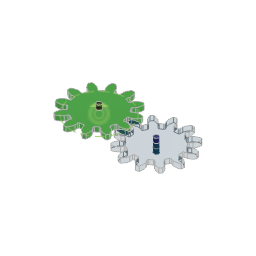
simple_gear_power (Autodesk Fusion 360 design; units mm, degrees)
description: Spur Gear; Module: 10.0; Num Teeth: 12; Pressure Angle: 20.0; Backlash: 0.00 mm
part number: 2026-04-30-14-06-16-626
part number: 2026-04-30-14-27-06-127
part number: 2026-04-30-14-27-10-473
part number: 2026-04-30-14-27-12-573
part number: 2026-04-30-14-27-14-794
Autodesk Fusion 360 part; units mm, degrees
(part 1 of 2)
sketch "Base Circle" plane through (0, 0, 0) normal (0, 0, 1) x (1, 0, 0)
  circle A0 centre (0, 0) radius 48.43
  circle A1 centre (0, 0) radius 5
extrude "Extrude5" add sketch "Base Circle" along normal blind 10 makes body 1
sketch "Gear Tooth" plane through (0, 0, 0) normal (0, 0, 1) x (1, 0, 0)
  spline S0 degree 5 poles (55.7833, -8.1916) (55.824, -8.1975) (55.9054, -8.2082) (56.0278, -8.2201) (56.1916, -8.2285) (56.3971, -8.2288) (56.6031, -8.2218) (56.8094, -8.2105) (57.0158, -8.1967) (57.2224, -8.1814) (57.429, -8.1642) (57.6357, -8.1445) (57.8425, -8.1217) (58.0493, -8.0952) (58.2562, -8.0651) (58.4632, -8.0317) (58.6701, -7.9955) (58.877, -7.957) (59.0839, -7.9164) (59.2907, -7.8739) (59.4973, -7.8293) (59.7039, -7.7827) (59.9104, -7.7337) (60.1168, -7.6825) (60.3231, -7.6291) (60.5293, -7.5736) (60.7353, -7.516) (60.9412, -7.4565) (61.1469, -7.3952) (61.3524, -7.332) (61.5578, -7.267) (61.7629, -7.2001) (61.9679, -7.1315) (62.1727, -7.061) (62.3773, -6.9888) (62.5816, -6.9148) (62.7857, -6.839) (62.9896, -6.7616) (63.1933, -6.6825) (63.3967, -6.6018) (63.5998, -6.5195) (63.8027, -6.4355) (64.0053, -6.3499) (64.2077, -6.2628) (64.4097, -6.174) (64.6115, -6.0837) (64.813, -5.9919) (65.0142, -5.8985) (65.2151, -5.8037) (65.4157, -5.7073) (65.616, -5.6095) (65.8159, -5.5101) (66.0155, -5.4094) (66.2148, -5.3071) (66.4138, -5.2035) (66.6124, -5.0984) (66.8106, -4.9919) (67.0085, -4.884) (67.2061, -4.7747) (67.4033, -4.664) (67.6001, -4.552) (67.7965, -4.4385) (67.9926, -4.3238) (68.1883, -4.2077) (68.3835, -4.0902) (68.5784, -3.9715) (68.7729, -3.8514) (68.967, -3.73) (69.1607, -3.6073) (69.354, -3.4834) (69.5468, -3.3581) (69.7008, -3.2569) (69.816, -3.1804) (69.8928, -3.1292) (69.9312, -3.1035) knots 0 0 0 0 0 0 0.01428571 0.02857143 0.04285714 0.05714286 0.07142857 0.08571429 0.1 0.11428571 0.12857143 0.14285714 0.15714286 0.17142857 0.18571429 0.2 0.21428571 0.22857143 0.24285714 0.25714286 0.27142857 0.28571429 0.3 0.31428571 0.32857143 0.34285714 0.35714286 0.37142857 0.38571429 0.4 0.41428571 0.42857143 0.44285714 0.45714286 0.47142857 0.48571429 0.5 0.51428571 0.52857143 0.54285714 0.55714286 0.57142857 0.58571429 0.6 0.61428571 0.62857143 0.64285714 0.65714286 0.67142857 0.68571429 0.7 0.71428571 0.72857143 0.74285714 0.75714286 0.77142857 0.78571429 0.8 0.81428571 0.82857143 0.84285714 0.85714286 0.87142857 0.88571429 0.9 0.91428571 0.92857143 0.94285714 0.95714286 0.97142857 0.98571429 1 1 1 1 1 1
  spline S1 degree 5 poles (55.7833, 8.1916) (55.824, 8.1975) (55.9054, 8.2082) (56.0278, 8.2201) (56.1916, 8.2285) (56.3971, 8.2288) (56.6031, 8.2218) (56.8094, 8.2105) (57.0158, 8.1967) (57.2224, 8.1814) (57.429, 8.1642) (57.6357, 8.1445) (57.8425, 8.1217) (58.0493, 8.0952) (58.2562, 8.0651) (58.4632, 8.0317) (58.6701, 7.9955) (58.877, 7.957) (59.0839, 7.9164) (59.2907, 7.8739) (59.4973, 7.8293) (59.7039, 7.7827) (59.9104, 7.7337) (60.1168, 7.6825) (60.3231, 7.6291) (60.5293, 7.5736) (60.7353, 7.516) (60.9412, 7.4565) (61.1469, 7.3952) (61.3524, 7.332) (61.5578, 7.267) (61.7629, 7.2001) (61.9679, 7.1315) (62.1727, 7.061) (62.3773, 6.9888) (62.5816, 6.9148) (62.7857, 6.839) (62.9896, 6.7616) (63.1933, 6.6825) (63.3967, 6.6018) (63.5998, 6.5195) (63.8027, 6.4355) (64.0053, 6.3499) (64.2077, 6.2628) (64.4097, 6.174) (64.6115, 6.0837) (64.813, 5.9919) (65.0142, 5.8985) (65.2151, 5.8037) (65.4157, 5.7073) (65.616, 5.6095) (65.8159, 5.5101) (66.0155, 5.4094) (66.2148, 5.3071) (66.4138, 5.2035) (66.6124, 5.0984) (66.8106, 4.9919) (67.0085, 4.884) (67.2061, 4.7747) (67.4033, 4.664) (67.6001, 4.552) (67.7965, 4.4385) (67.9926, 4.3238) (68.1883, 4.2077) (68.3835, 4.0902) (68.5784, 3.9715) (68.7729, 3.8514) (68.967, 3.73) (69.1607, 3.6073) (69.354, 3.4834) (69.5468, 3.3581) (69.7008, 3.2569) (69.816, 3.1804) (69.8928, 3.1292) (69.9312, 3.1035) knots 0 0 0 0 0 0 0.01428571 0.02857143 0.04285714 0.05714286 0.07142857 0.08571429 0.1 0.11428571 0.12857143 0.14285714 0.15714286 0.17142857 0.18571429 0.2 0.21428571 0.22857143 0.24285714 0.25714286 0.27142857 0.28571429 0.3 0.31428571 0.32857143 0.34285714 0.35714286 0.37142857 0.38571429 0.4 0.41428571 0.42857143 0.44285714 0.45714286 0.47142857 0.48571429 0.5 0.51428571 0.52857143 0.54285714 0.55714286 0.57142857 0.58571429 0.6 0.61428571 0.62857143 0.64285714 0.65714286 0.67142857 0.68571429 0.7 0.71428571 0.72857143 0.74285714 0.75714286 0.77142857 0.78571429 0.8 0.81428571 0.82857143 0.84285714 0.85714286 0.87142857 0.88571429 0.9 0.91428571 0.92857143 0.94285714 0.95714286 0.97142857 0.98571429 1 1 1 1 1 1
  arc A0 (69.9312, -3.1035) -> (69.9312, 3.1035) centre (0, 0) ccw
  line L0 (47.9062, -7.0348) -> (55.7833, -8.1916)
  line L1 (47.9062, 7.0348) -> (55.7833, 8.1916)
  line L2 (47.9062, -7.0348) -> (47.9062, 7.0348)
  point P0 (56.7633, -8.2126)
  point P1 (57.7576, -8.1306)
  point P2 (58.7606, -7.9784)
  point P3 (59.77, -7.7667)
  point P4 (60.7841, -7.5016)
  point P5 (61.8016, -7.1869)
  point P6 (62.8211, -6.8253)
  point P7 (63.8417, -6.4188)
  point P8 (64.8622, -5.9688)
  point P9 (65.8818, -5.4767)
  point P10 (66.8994, -4.9433)
  point P11 (67.9141, -4.3695)
  point P12 (68.925, -3.756)
  point P13 (56.7633, 8.2126)
  point P14 (57.7576, 8.1306)
  point P15 (58.7606, 7.9784)
  point P16 (59.77, 7.7667)
  point P17 (60.7841, 7.5016)
  point P18 (61.8016, 7.1869)
  point P19 (62.8211, 6.8253)
  point P20 (63.8417, 6.4188)
  point P21 (64.8622, 5.9688)
  point P22 (65.8818, 5.4767)
  point P23 (66.8994, 4.9433)
  point P24 (67.9141, 4.3695)
  point P25 (68.925, 3.756)
extrude "Extrude6" add sketch "Gear Tooth" along normal blind 10 bodies 1
fillet "Fillet3" radius 2 2 edges at (47.9161, -7.0363, 5) (47.9161, 7.0363, 5) on bodies 1
pattern_circular "C-Pattern3" count 12 over 360 about axis through (0, 0, 0) along (0, 0, 1) of "Extrude6", "Fillet3"
sketch "Diametrial Pitch Circle" plane through (0, 0, 0) normal (0, 0, 1) x (1, 0, 0)
  circle A0 centre (0, 0) radius 60 construction
sketch "Base Circle (1)" plane through (0, 0, 0) normal (0, 0, 1) x (1, 0, 0)
  circle A0 centre (0, 0) radius 48.43
  circle A1 centre (0, 0) radius 5
extrude "Extrude7" add sketch "Base Circle (1)" along normal blind 10 separate body makes body 2
sketch "Gear Tooth (1)" plane through (0, 0, 0) normal (0, 0, 1) x (1, 0, 0)
  spline S0 degree 5 poles (55.7833, -8.1916) (55.824, -8.1975) (55.9054, -8.2082) (56.0278, -8.2201) (56.1916, -8.2285) (56.3971, -8.2288) (56.6031, -8.2218) (56.8094, -8.2105) (57.0158, -8.1967) (57.2224, -8.1814) (57.429, -8.1642) (57.6357, -8.1445) (57.8425, -8.1217) (58.0493, -8.0952) (58.2562, -8.0651) (58.4632, -8.0317) (58.6701, -7.9955) (58.877, -7.957) (59.0839, -7.9164) (59.2907, -7.8739) (59.4973, -7.8293) (59.7039, -7.7827) (59.9104, -7.7337) (60.1168, -7.6825) (60.3231, -7.6291) (60.5293, -7.5736) (60.7353, -7.516) (60.9412, -7.4565) (61.1469, -7.3952) (61.3524, -7.332) (61.5578, -7.267) (61.7629, -7.2001) (61.9679, -7.1315) (62.1727, -7.061) (62.3773, -6.9888) (62.5816, -6.9148) (62.7857, -6.839) (62.9896, -6.7616) (63.1933, -6.6825) (63.3967, -6.6018) (63.5998, -6.5195) (63.8027, -6.4355) (64.0053, -6.3499) (64.2077, -6.2628) (64.4097, -6.174) (64.6115, -6.0837) (64.813, -5.9919) (65.0142, -5.8985) (65.2151, -5.8037) (65.4157, -5.7073) (65.616, -5.6095) (65.8159, -5.5101) (66.0155, -5.4094) (66.2148, -5.3071) (66.4138, -5.2035) (66.6124, -5.0984) (66.8106, -4.9919) (67.0085, -4.884) (67.2061, -4.7747) (67.4033, -4.664) (67.6001, -4.552) (67.7965, -4.4385) (67.9926, -4.3238) (68.1883, -4.2077) (68.3835, -4.0902) (68.5784, -3.9715) (68.7729, -3.8514) (68.967, -3.73) (69.1607, -3.6073) (69.354, -3.4834) (69.5468, -3.3581) (69.7008, -3.2569) (69.816, -3.1804) (69.8928, -3.1292) (69.9312, -3.1035) knots 0 0 0 0 0 0 0.01428571 0.02857143 0.04285714 0.05714286 0.07142857 0.08571429 0.1 0.11428571 0.12857143 0.14285714 0.15714286 0.17142857 0.18571429 0.2 0.21428571 0.22857143 0.24285714 0.25714286 0.27142857 0.28571429 0.3 0.31428571 0.32857143 0.34285714 0.35714286 0.37142857 0.38571429 0.4 0.41428571 0.42857143 0.44285714 0.45714286 0.47142857 0.48571429 0.5 0.51428571 0.52857143 0.54285714 0.55714286 0.57142857 0.58571429 0.6 0.61428571 0.62857143 0.64285714 0.65714286 0.67142857 0.68571429 0.7 0.71428571 0.72857143 0.74285714 0.75714286 0.77142857 0.78571429 0.8 0.81428571 0.82857143 0.84285714 0.85714286 0.87142857 0.88571429 0.9 0.91428571 0.92857143 0.94285714 0.95714286 0.97142857 0.98571429 1 1 1 1 1 1
  spline S1 degree 5 poles (55.7833, 8.1916) (55.824, 8.1975) (55.9054, 8.2082) (56.0278, 8.2201) (56.1916, 8.2285) (56.3971, 8.2288) (56.6031, 8.2218) (56.8094, 8.2105) (57.0158, 8.1967) (57.2224, 8.1814) (57.429, 8.1642) (57.6357, 8.1445) (57.8425, 8.1217) (58.0493, 8.0952) (58.2562, 8.0651) (58.4632, 8.0317) (58.6701, 7.9955) (58.877, 7.957) (59.0839, 7.9164) (59.2907, 7.8739) (59.4973, 7.8293) (59.7039, 7.7827) (59.9104, 7.7337) (60.1168, 7.6825) (60.3231, 7.6291) (60.5293, 7.5736) (60.7353, 7.516) (60.9412, 7.4565) (61.1469, 7.3952) (61.3524, 7.332) (61.5578, 7.267) (61.7629, 7.2001) (61.9679, 7.1315) (62.1727, 7.061) (62.3773, 6.9888) (62.5816, 6.9148) (62.7857, 6.839) (62.9896, 6.7616) (63.1933, 6.6825) (63.3967, 6.6018) (63.5998, 6.5195) (63.8027, 6.4355) (64.0053, 6.3499) (64.2077, 6.2628) (64.4097, 6.174) (64.6115, 6.0837) (64.813, 5.9919) (65.0142, 5.8985) (65.2151, 5.8037) (65.4157, 5.7073) (65.616, 5.6095) (65.8159, 5.5101) (66.0155, 5.4094) (66.2148, 5.3071) (66.4138, 5.2035) (66.6124, 5.0984) (66.8106, 4.9919) (67.0085, 4.884) (67.2061, 4.7747) (67.4033, 4.664) (67.6001, 4.552) (67.7965, 4.4385) (67.9926, 4.3238) (68.1883, 4.2077) (68.3835, 4.0902) (68.5784, 3.9715) (68.7729, 3.8514) (68.967, 3.73) (69.1607, 3.6073) (69.354, 3.4834) (69.5468, 3.3581) (69.7008, 3.2569) (69.816, 3.1804) (69.8928, 3.1292) (69.9312, 3.1035) knots 0 0 0 0 0 0 0.01428571 0.02857143 0.04285714 0.05714286 0.07142857 0.08571429 0.1 0.11428571 0.12857143 0.14285714 0.15714286 0.17142857 0.18571429 0.2 0.21428571 0.22857143 0.24285714 0.25714286 0.27142857 0.28571429 0.3 0.31428571 0.32857143 0.34285714 0.35714286 0.37142857 0.38571429 0.4 0.41428571 0.42857143 0.44285714 0.45714286 0.47142857 0.48571429 0.5 0.51428571 0.52857143 0.54285714 0.55714286 0.57142857 0.58571429 0.6 0.61428571 0.62857143 0.64285714 0.65714286 0.67142857 0.68571429 0.7 0.71428571 0.72857143 0.74285714 0.75714286 0.77142857 0.78571429 0.8 0.81428571 0.82857143 0.84285714 0.85714286 0.87142857 0.88571429 0.9 0.91428571 0.92857143 0.94285714 0.95714286 0.97142857 0.98571429 1 1 1 1 1 1
  arc A0 (69.9312, -3.1035) -> (69.9312, 3.1035) centre (0, 0) ccw
  line L0 (47.9062, -7.0348) -> (55.7833, -8.1916)
  line L1 (47.9062, 7.0348) -> (55.7833, 8.1916)
  line L2 (47.9062, -7.0348) -> (47.9062, 7.0348)
  point P0 (56.7633, -8.2126)
  point P1 (57.7576, -8.1306)
  point P2 (58.7606, -7.9784)
  point P3 (59.77, -7.7667)
  point P4 (60.7841, -7.5016)
  point P5 (61.8016, -7.1869)
  point P6 (62.8211, -6.8253)
  point P7 (63.8417, -6.4188)
  point P8 (64.8622, -5.9688)
  point P9 (65.8818, -5.4767)
  point P10 (66.8994, -4.9433)
  point P11 (67.9141, -4.3695)
  point P12 (68.925, -3.756)
  point P13 (56.7633, 8.2126)
  point P14 (57.7576, 8.1306)
  point P15 (58.7606, 7.9784)
  point P16 (59.77, 7.7667)
  point P17 (60.7841, 7.5016)
  point P18 (61.8016, 7.1869)
  point P19 (62.8211, 6.8253)
  point P20 (63.8417, 6.4188)
  point P21 (64.8622, 5.9688)
  point P22 (65.8818, 5.4767)
  point P23 (66.8994, 4.9433)
  point P24 (67.9141, 4.3695)
  point P25 (68.925, 3.756)
extrude "Extrude8" add sketch "Gear Tooth (1)" along normal blind 10 bodies 2
fillet "Fillet4" radius 2 2 edges at (47.9161, -7.0363, 5) (47.9161, 7.0363, 5) on bodies 2
pattern_circular "C-Pattern4" count 12 over 360 about axis through (0, 0, 0) along (0, 0, 1) of "Extrude8", "Fillet4"
sketch "Diametrial Pitch Circle (1)" plane through (0, 0, 0) normal (0, 0, 1) x (1, 0, 0)
  circle A0 centre (0, 0) radius 60 construction
move_body "Move1" bodies 2 to x (1, 0, 0) y (0, 1, 0) z (0, 0, 1) at (120, 0, 0)
sketch "Sketch14" plane through (0, 0, 10) normal (0, 0, 1) x (-1, 0, 0)
  arc A0 (-45.6878, 16.0652) -> (-47.5994, 8.9311) centre (0, 0) ccw
  arc A1 (-49.8557, 7.3211) -> (-47.5994, 8.9311) centre (-49.5651, 9.2999) ccw
  line L0 (-49.8557, 7.3211) -> (-55.7833, 8.1916)
  spline S0 degree 5 poles (-55.7833, 8.1916) (-55.824, 8.1975) (-55.9054, 8.2082) (-56.0278, 8.2201) (-56.1916, 8.2285) (-56.3971, 8.2288) (-56.6031, 8.2218) (-56.8094, 8.2105) (-57.0158, 8.1967) (-57.2224, 8.1814) (-57.429, 8.1642) (-57.6357, 8.1445) (-57.8425, 8.1217) (-58.0493, 8.0952) (-58.2562, 8.0651) (-58.4632, 8.0317) (-58.6701, 7.9955) (-58.877, 7.957) (-59.0839, 7.9164) (-59.2907, 7.8739) (-59.4973, 7.8293) (-59.7039, 7.7827) (-59.9104, 7.7337) (-60.1168, 7.6825) (-60.3231, 7.6291) (-60.5293, 7.5736) (-60.7353, 7.516) (-60.9412, 7.4565) (-61.1469, 7.3952) (-61.3524, 7.332) (-61.5578, 7.267) (-61.7629, 7.2001) (-61.9679, 7.1315) (-62.1727, 7.061) (-62.3773, 6.9888) (-62.5816, 6.9148) (-62.7857, 6.839) (-62.9896, 6.7616) (-63.1933, 6.6825) (-63.3967, 6.6018) (-63.5998, 6.5195) (-63.8027, 6.4355) (-64.0053, 6.3499) (-64.2077, 6.2628) (-64.4097, 6.174) (-64.6115, 6.0837) (-64.813, 5.9919) (-65.0142, 5.8985) (-65.2151, 5.8037) (-65.4157, 5.7073) (-65.616, 5.6095) (-65.8159, 5.5101) (-66.0155, 5.4094) (-66.2148, 5.3071) (-66.4138, 5.2035) (-66.6124, 5.0984) (-66.8106, 4.9919) (-67.0085, 4.884) (-67.2061, 4.7747) (-67.4033, 4.664) (-67.6001, 4.552) (-67.7965, 4.4385) (-67.9926, 4.3238) (-68.1883, 4.2077) (-68.3835, 4.0902) (-68.5784, 3.9715) (-68.7729, 3.8514) (-68.967, 3.73) (-69.1607, 3.6073) (-69.354, 3.4834) (-69.5468, 3.3581) (-69.7008, 3.2569) (-69.816, 3.1804) (-69.8928, 3.1292) (-69.9312, 3.1035) knots 0 0 0 0 0 0 0.01428571 0.02857143 0.04285714 0.05714286 0.07142857 0.08571429 0.1 0.11428571 0.12857143 0.14285714 0.15714286 0.17142857 0.18571429 0.2 0.21428571 0.22857143 0.24285714 0.25714286 0.27142857 0.28571429 0.3 0.31428571 0.32857143 0.34285714 0.35714286 0.37142857 0.38571429 0.4 0.41428571 0.42857143 0.44285714 0.45714286 0.47142857 0.48571429 0.5 0.51428571 0.52857143 0.54285714 0.55714286 0.57142857 0.58571429 0.6 0.61428571 0.62857143 0.64285714 0.65714286 0.67142857 0.68571429 0.7 0.71428571 0.72857143 0.74285714 0.75714286 0.77142857 0.78571429 0.8 0.81428571 0.82857143 0.84285714 0.85714286 0.87142857 0.88571429 0.9 0.91428571 0.92857143 0.94285714 0.95714286 0.97142857 0.98571429 1 1 1 1 1 1
  arc A2 (-69.9312, 3.1035) -> (-69.9312, -3.1035) centre (0, 0) ccw
  spline S1 degree 5 poles (-69.9312, -3.1035) (-69.8928, -3.1292) (-69.816, -3.1804) (-69.7008, -3.2569) (-69.5468, -3.3581) (-69.354, -3.4834) (-69.1607, -3.6073) (-68.967, -3.73) (-68.7729, -3.8514) (-68.5784, -3.9715) (-68.3835, -4.0902) (-68.1883, -4.2077) (-67.9926, -4.3238) (-67.7965, -4.4385) (-67.6001, -4.552) (-67.4033, -4.664) (-67.2061, -4.7747) (-67.0085, -4.884) (-66.8106, -4.9919) (-66.6124, -5.0984) (-66.4138, -5.2035) (-66.2148, -5.3071) (-66.0155, -5.4094) (-65.8159, -5.5101) (-65.616, -5.6095) (-65.4157, -5.7073) (-65.2151, -5.8037) (-65.0142, -5.8985) (-64.813, -5.9919) (-64.6115, -6.0837) (-64.4097, -6.174) (-64.2077, -6.2628) (-64.0053, -6.3499) (-63.8027, -6.4355) (-63.5998, -6.5195) (-63.3967, -6.6018) (-63.1933, -6.6825) (-62.9896, -6.7616) (-62.7857, -6.839) (-62.5816, -6.9148) (-62.3773, -6.9888) (-62.1727, -7.061) (-61.9679, -7.1315) (-61.7629, -7.2001) (-61.5578, -7.267) (-61.3524, -7.332) (-61.1469, -7.3952) (-60.9412, -7.4565) (-60.7353, -7.516) (-60.5293, -7.5736) (-60.3231, -7.6291) (-60.1168, -7.6825) (-59.9104, -7.7337) (-59.7039, -7.7827) (-59.4973, -7.8293) (-59.2907, -7.8739) (-59.0839, -7.9164) (-58.877, -7.957) (-58.6701, -7.9955) (-58.4632, -8.0317) (-58.2562, -8.0651) (-58.0493, -8.0952) (-57.8425, -8.1217) (-57.6357, -8.1445) (-57.429, -8.1642) (-57.2224, -8.1814) (-57.0158, -8.1967) (-56.8094, -8.2105) (-56.6031, -8.2218) (-56.3971, -8.2288) (-56.1916, -8.2285) (-56.0278, -8.2201) (-55.9054, -8.2082) (-55.824, -8.1975) (-55.7833, -8.1916) knots -1 -1 -1 -1 -1 -1 -0.98571429 -0.97142857 -0.95714286 -0.94285714 -0.92857143 -0.91428571 -0.9 -0.88571429 -0.87142857 -0.85714286 -0.84285714 -0.82857143 -0.81428571 -0.8 -0.78571429 -0.77142857 -0.75714286 -0.74285714 -0.72857143 -0.71428571 -0.7 -0.68571429 -0.67142857 -0.65714286 -0.64285714 -0.62857143 -0.61428571 -0.6 -0.58571429 -0.57142857 -0.55714286 -0.54285714 -0.52857143 -0.51428571 -0.5 -0.48571429 -0.47142857 -0.45714286 -0.44285714 -0.42857143 -0.41428571 -0.4 -0.38571429 -0.37142857 -0.35714286 -0.34285714 -0.32857143 -0.31428571 -0.3 -0.28571429 -0.27142857 -0.25714286 -0.24285714 -0.22857143 -0.21428571 -0.2 -0.18571429 -0.17142857 -0.15714286 -0.14285714 -0.12857143 -0.11428571 -0.1 -0.08571429 -0.07142857 -0.05714286 -0.04285714 -0.02857143 -0.01428571 0 0 0 0 0 0
  line L1 (-55.7833, -8.1916) -> (-49.8557, -7.3211)
  arc A3 (-47.5994, -8.9311) -> (-49.8557, -7.3211) centre (-49.5651, -9.2999) ccw
  arc A4 (-47.5994, -8.9311) -> (-45.6878, -16.0652) centre (0, 0) ccw
  arc A5 (-46.8368, -18.5876) -> (-45.6878, -16.0652) centre (-47.5746, -16.7286) ccw
  line L2 (-46.8368, -18.5876) -> (-52.4056, -20.7976)
  spline S2 degree 5 poles (-52.4056, -20.7976) (-52.4438, -20.8127) (-52.5196, -20.8442) (-52.6316, -20.8951) (-52.7776, -20.9697) (-52.9557, -21.0722) (-53.1306, -21.1812) (-53.3036, -21.2942) (-53.4755, -21.4093) (-53.6467, -21.5259) (-53.8171, -21.6441) (-53.9863, -21.7645) (-54.1539, -21.8876) (-54.3198, -22.014) (-54.4839, -22.1436) (-54.6464, -22.276) (-54.8076, -22.4108) (-54.9675, -22.5476) (-55.1264, -22.6861) (-55.2842, -22.8264) (-55.4409, -22.9683) (-55.5965, -23.112) (-55.7508, -23.2576) (-55.904, -23.4052) (-56.0559, -23.5546) (-56.2067, -23.7057) (-56.3563, -23.8586) (-56.5049, -24.0131) (-56.6523, -24.1691) (-56.7987, -24.3265) (-56.9441, -24.4855) (-57.0884, -24.646) (-57.2315, -24.8079) (-57.3736, -24.9713) (-57.5147, -25.1362) (-57.6546, -25.3024) (-57.7936, -25.4701) (-57.9314, -25.6391) (-58.0682, -25.8094) (-58.204, -25.981) (-58.3388, -26.1539) (-58.4725, -26.328) (-58.6052, -26.5035) (-58.7369, -26.6801) (-58.8675, -26.858) (-58.9971, -27.0371) (-59.1257, -27.2174) (-59.2532, -27.3988) (-59.3798, -27.5814) (-59.5053, -27.7652) (-59.6298, -27.95) (-59.7533, -28.136) (-59.8758, -28.3231) (-59.9973, -28.5113) (-60.1177, -28.7005) (-60.2372, -28.8909) (-60.3556, -29.0822) (-60.4731, -29.2746) (-60.5895, -29.468) (-60.7049, -29.6625) (-60.8194, -29.8579) (-60.9328, -30.0544) (-61.0452, -30.2518) (-61.1566, -30.4502) (-61.267, -30.6495) (-61.3764, -30.8498) (-61.4848, -31.0511) (-61.5922, -31.2532) (-61.6986, -31.4563) (-61.804, -31.6603) (-61.9084, -31.8652) (-61.9911, -32.0298) (-62.0527, -32.1537) (-62.0935, -32.2365) (-62.1139, -32.2779) knots 0 0 0 0 0 0 0.01428571 0.02857143 0.04285714 0.05714286 0.07142857 0.08571429 0.1 0.11428571 0.12857143 0.14285714 0.15714286 0.17142857 0.18571429 0.2 0.21428571 0.22857143 0.24285714 0.25714286 0.27142857 0.28571429 0.3 0.31428571 0.32857143 0.34285714 0.35714286 0.37142857 0.38571429 0.4 0.41428571 0.42857143 0.44285714 0.45714286 0.47142857 0.48571429 0.5 0.51428571 0.52857143 0.54285714 0.55714286 0.57142857 0.58571429 0.6 0.61428571 0.62857143 0.64285714 0.65714286 0.67142857 0.68571429 0.7 0.71428571 0.72857143 0.74285714 0.75714286 0.77142857 0.78571429 0.8 0.81428571 0.82857143 0.84285714 0.85714286 0.87142857 0.88571429 0.9 0.91428571 0.92857143 0.94285714 0.95714286 0.97142857 0.98571429 1 1 1 1 1 1
  arc A6 (-62.1139, -32.2779) -> (-59.0104, -37.6533) centre (0, 0) ccw
  spline S3 degree 5 poles (-59.0104, -37.6533) (-58.9644, -37.6563) (-58.8723, -37.6623) (-58.7342, -37.6709) (-58.5502, -37.6816) (-58.3206, -37.6937) (-58.0913, -37.7044) (-57.8622, -37.7138) (-57.6334, -37.7219) (-57.4049, -37.7286) (-57.1768, -37.734) (-56.9489, -37.7381) (-56.7214, -37.7408) (-56.4942, -37.7421) (-56.2674, -37.7421) (-56.0409, -37.7408) (-55.8148, -37.738) (-55.5891, -37.7339) (-55.3638, -37.7284) (-55.1388, -37.7215) (-54.9143, -37.7132) (-54.6901, -37.7035) (-54.4664, -37.6924) (-54.2432, -37.6799) (-54.0204, -37.6659) (-53.798, -37.6505) (-53.5761, -37.6337) (-53.3547, -37.6154) (-53.1338, -37.5957) (-52.9134, -37.5744) (-52.6935, -37.5517) (-52.4741, -37.5276) (-52.2553, -37.5019) (-52.037, -37.4747) (-51.8193, -37.4459) (-51.6022, -37.4157) (-51.3857, -37.3839) (-51.1698, -37.3505) (-50.9545, -37.3156) (-50.7399, -37.2792) (-50.5259, -37.2411) (-50.3126, -37.2014) (-50.1, -37.16) (-49.8882, -37.117) (-49.6771, -37.0723) (-49.4668, -37.0259) (-49.2572, -36.9778) (-49.0484, -36.9281) (-48.8403, -36.8767) (-48.6331, -36.8235) (-48.4268, -36.7686) (-48.2214, -36.7117) (-48.0171, -36.6528) (-47.8138, -36.5919) (-47.6115, -36.5291) (-47.4103, -36.4643) (-47.2099, -36.3978) (-47.0105, -36.3295) (-46.8121, -36.2594) (-46.6148, -36.1872) (-46.4188, -36.1127) (-46.2246, -36.0353) (-46.0322, -35.9548) (-45.8417, -35.8712) (-45.6529, -35.7849) (-45.4654, -35.6965) (-45.2788, -35.6065) (-45.0931, -35.5151) (-44.9088, -35.4218) (-44.7269, -35.3249) (-44.5491, -35.2219) (-44.4115, -35.1327) (-44.3114, -35.0612) (-44.2462, -35.0113) (-44.214, -34.9858) knots -1 -1 -1 -1 -1 -1 -0.98571429 -0.97142857 -0.95714286 -0.94285714 -0.92857143 -0.91428571 -0.9 -0.88571429 -0.87142857 -0.85714286 -0.84285714 -0.82857143 -0.81428571 -0.8 -0.78571429 -0.77142857 -0.75714286 -0.74285714 -0.72857143 -0.71428571 -0.7 -0.68571429 -0.67142857 -0.65714286 -0.64285714 -0.62857143 -0.61428571 -0.6 -0.58571429 -0.57142857 -0.55714286 -0.54285714 -0.52857143 -0.51428571 -0.5 -0.48571429 -0.47142857 -0.45714286 -0.44285714 -0.42857143 -0.41428571 -0.4 -0.38571429 -0.37142857 -0.35714286 -0.34285714 -0.32857143 -0.31428571 -0.3 -0.28571429 -0.27142857 -0.25714286 -0.24285714 -0.22857143 -0.21428571 -0.2 -0.18571429 -0.17142857 -0.15714286 -0.14285714 -0.12857143 -0.11428571 -0.1 -0.08571429 -0.07142857 -0.05714286 -0.04285714 -0.02857143 -0.01428571 0 0 0 0 0 0
  line L3 (-44.214, -34.9858) -> (-39.5157, -31.2681)
  arc A7 (-36.7567, -31.5342) -> (-39.5157, -31.2681) centre (-38.2747, -32.8365) ccw
  arc A8 (-36.7567, -31.5342) -> (-31.5342, -36.7567) centre (0, 0) ccw
  arc A9 (-31.2681, -39.5157) -> (-31.5342, -36.7567) centre (-32.8365, -38.2747) ccw
  line L4 (-31.2681, -39.5157) -> (-34.9858, -44.214)
  spline S4 degree 5 poles (-34.9858, -44.214) (-35.0113, -44.2462) (-35.0612, -44.3114) (-35.1327, -44.4115) (-35.2219, -44.5491) (-35.3249, -44.7269) (-35.4218, -44.9088) (-35.5151, -45.0931) (-35.6065, -45.2788) (-35.6965, -45.4654) (-35.7849, -45.6529) (-35.8712, -45.8417) (-35.9548, -46.0322) (-36.0353, -46.2246) (-36.1127, -46.4188) (-36.1872, -46.6148) (-36.2594, -46.8121) (-36.3295, -47.0105) (-36.3978, -47.2099) (-36.4643, -47.4103) (-36.5291, -47.6115) (-36.5919, -47.8138) (-36.6528, -48.0171) (-36.7117, -48.2214) (-36.7686, -48.4268) (-36.8235, -48.6331) (-36.8767, -48.8403) (-36.9281, -49.0484) (-36.9778, -49.2572) (-37.0259, -49.4668) (-37.0723, -49.6771) (-37.117, -49.8882) (-37.16, -50.1) (-37.2014, -50.3126) (-37.2411, -50.5259) (-37.2792, -50.7399) (-37.3156, -50.9545) (-37.3505, -51.1698) (-37.3839, -51.3857) (-37.4157, -51.6022) (-37.4459, -51.8193) (-37.4747, -52.037) (-37.5019, -52.2553) (-37.5276, -52.4741) (-37.5517, -52.6935) (-37.5744, -52.9134) (-37.5957, -53.1338) (-37.6154, -53.3547) (-37.6337, -53.5761) (-37.6505, -53.798) (-37.6659, -54.0204) (-37.6799, -54.2432) (-37.6924, -54.4664) (-37.7035, -54.6901) (-37.7132, -54.9143) (-37.7215, -55.1388) (-37.7284, -55.3638) (-37.7339, -55.5891) (-37.738, -55.8148) (-37.7408, -56.0409) (-37.7421, -56.2674) (-37.7421, -56.4942) (-37.7408, -56.7214) (-37.7381, -56.9489) (-37.734, -57.1768) (-37.7286, -57.4049) (-37.7219, -57.6334) (-37.7138, -57.8622) (-37.7044, -58.0913) (-37.6937, -58.3206) (-37.6816, -58.5502) (-37.6709, -58.7342) (-37.6623, -58.8723) (-37.6563, -58.9644) (-37.6533, -59.0104) knots 0 0 0 0 0 0 0.01428571 0.02857143 0.04285714 0.05714286 0.07142857 0.08571429 0.1 0.11428571 0.12857143 0.14285714 0.15714286 0.17142857 0.18571429 0.2 0.21428571 0.22857143 0.24285714 0.25714286 0.27142857 0.28571429 0.3 0.31428571 0.32857143 0.34285714 0.35714286 0.37142857 0.38571429 0.4 0.41428571 0.42857143 0.44285714 0.45714286 0.47142857 0.48571429 0.5 0.51428571 0.52857143 0.54285714 0.55714286 0.57142857 0.58571429 0.6 0.61428571 0.62857143 0.64285714 0.65714286 0.67142857 0.68571429 0.7 0.71428571 0.72857143 0.74285714 0.75714286 0.77142857 0.78571429 0.8 0.81428571 0.82857143 0.84285714 0.85714286 0.87142857 0.88571429 0.9 0.91428571 0.92857143 0.94285714 0.95714286 0.97142857 0.98571429 1 1 1 1 1 1
  arc A10 (-37.6533, -59.0104) -> (-32.2779, -62.1139) centre (0, 0) ccw
  spline S5 degree 5 poles (-32.2779, -62.1139) (-32.2365, -62.0935) (-32.1537, -62.0527) (-32.0298, -61.9911) (-31.8652, -61.9084) (-31.6603, -61.804) (-31.4563, -61.6986) (-31.2532, -61.5922) (-31.0511, -61.4848) (-30.8498, -61.3764) (-30.6495, -61.267) (-30.4502, -61.1566) (-30.2518, -61.0452) (-30.0544, -60.9328) (-29.8579, -60.8194) (-29.6625, -60.7049) (-29.468, -60.5895) (-29.2746, -60.4731) (-29.0822, -60.3556) (-28.8909, -60.2372) (-28.7005, -60.1177) (-28.5113, -59.9973) (-28.3231, -59.8758) (-28.136, -59.7533) (-27.95, -59.6298) (-27.7652, -59.5053) (-27.5814, -59.3798) (-27.3988, -59.2532) (-27.2174, -59.1257) (-27.0371, -58.9971) (-26.858, -58.8675) (-26.6801, -58.7369) (-26.5035, -58.6052) (-26.328, -58.4725) (-26.1539, -58.3388) (-25.981, -58.204) (-25.8094, -58.0682) (-25.6391, -57.9314) (-25.4701, -57.7936) (-25.3024, -57.6546) (-25.1362, -57.5147) (-24.9713, -57.3736) (-24.8079, -57.2315) (-24.646, -57.0884) (-24.4855, -56.9441) (-24.3265, -56.7987) (-24.1691, -56.6523) (-24.0131, -56.5049) (-23.8586, -56.3563) (-23.7057, -56.2067) (-23.5546, -56.0559) (-23.4052, -55.904) (-23.2576, -55.7508) (-23.112, -55.5965) (-22.9683, -55.4409) (-22.8264, -55.2842) (-22.6861, -55.1264) (-22.5476, -54.9675) (-22.4108, -54.8076) (-22.276, -54.6464) (-22.1436, -54.4839) (-22.014, -54.3198) (-21.8876, -54.1539) (-21.7645, -53.9863) (-21.6441, -53.8171) (-21.5259, -53.6467) (-21.4093, -53.4755) (-21.2942, -53.3036) (-21.1812, -53.1306) (-21.0722, -52.9557) (-20.9697, -52.7776) (-20.8951, -52.6316) (-20.8442, -52.5196) (-20.8127, -52.4438) (-20.7976, -52.4056) knots -1 -1 -1 -1 -1 -1 -0.98571429 -0.97142857 -0.95714286 -0.94285714 -0.92857143 -0.91428571 -0.9 -0.88571429 -0.87142857 -0.85714286 -0.84285714 -0.82857143 -0.81428571 -0.8 -0.78571429 -0.77142857 -0.75714286 -0.74285714 -0.72857143 -0.71428571 -0.7 -0.68571429 -0.67142857 -0.65714286 -0.64285714 -0.62857143 -0.61428571 -0.6 -0.58571429 -0.57142857 -0.55714286 -0.54285714 -0.52857143 -0.51428571 -0.5 -0.48571429 -0.47142857 -0.45714286 -0.44285714 -0.42857143 -0.41428571 -0.4 -0.38571429 -0.37142857 -0.35714286 -0.34285714 -0.32857143 -0.31428571 -0.3 -0.28571429 -0.27142857 -0.25714286 -0.24285714 -0.22857143 -0.21428571 -0.2 -0.18571429 -0.17142857 -0.15714286 -0.14285714 -0.12857143 -0.11428571 -0.1 -0.08571429 -0.07142857 -0.05714286 -0.04285714 -0.02857143 -0.01428571 0 0 0 0 0 0
  line L5 (-20.7976, -52.4056) -> (-18.5876, -46.8368)
  arc A11 (-16.0652, -45.6878) -> (-18.5876, -46.8368) centre (-16.7286, -47.5746) ccw
  arc A12 (-16.0652, -45.6878) -> (-8.9311, -47.5994) centre (0, 0) ccw
  arc A13 (-7.3211, -49.8557) -> (-8.9311, -47.5994) centre (-9.2999, -49.5651) ccw
  line L6 (-7.3211, -49.8557) -> (-8.1916, -55.7833)
  spline S6 degree 5 poles (-8.1916, -55.7833) (-8.1975, -55.824) (-8.2082, -55.9054) (-8.2201, -56.0278) (-8.2285, -56.1916) (-8.2288, -56.3971) (-8.2218, -56.6031) (-8.2105, -56.8094) (-8.1967, -57.0158) (-8.1814, -57.2224) (-8.1642, -57.429) (-8.1445, -57.6357) (-8.1217, -57.8425) (-8.0952, -58.0493) (-8.0651, -58.2562) (-8.0317, -58.4632) (-7.9955, -58.6701) (-7.957, -58.877) (-7.9164, -59.0839) (-7.8739, -59.2907) (-7.8293, -59.4973) (-7.7827, -59.7039) (-7.7337, -59.9104) (-7.6825, -60.1168) (-7.6291, -60.3231) (-7.5736, -60.5293) (-7.516, -60.7353) (-7.4565, -60.9412) (-7.3952, -61.1469) (-7.332, -61.3524) (-7.267, -61.5578) (-7.2001, -61.7629) (-7.1315, -61.9679) (-7.061, -62.1727) (-6.9888, -62.3773) (-6.9148, -62.5816) (-6.839, -62.7857) (-6.7616, -62.9896) (-6.6825, -63.1933) (-6.6018, -63.3967) (-6.5195, -63.5998) (-6.4355, -63.8027) (-6.3499, -64.0053) (-6.2628, -64.2077) (-6.174, -64.4097) (-6.0837, -64.6115) (-5.9919, -64.813) (-5.8985, -65.0142) (-5.8037, -65.2151) (-5.7073, -65.4157) (-5.6095, -65.616) (-5.5101, -65.8159) (-5.4094, -66.0155) (-5.3071, -66.2148) (-5.2035, -66.4138) (-5.0984, -66.6124) (-4.9919, -66.8106) (-4.884, -67.0085) (-4.7747, -67.2061) (-4.664, -67.4033) (-4.552, -67.6001) (-4.4385, -67.7965) (-4.3238, -67.9926) (-4.2077, -68.1883) (-4.0902, -68.3835) (-3.9715, -68.5784) (-3.8514, -68.7729) (-3.73, -68.967) (-3.6073, -69.1607) (-3.4834, -69.354) (-3.3581, -69.5468) (-3.2569, -69.7008) (-3.1804, -69.816) (-3.1292, -69.8928) (-3.1035, -69.9312) knots 0 0 0 0 0 0 0.01428571 0.02857143 0.04285714 0.05714286 0.07142857 0.08571429 0.1 0.11428571 0.12857143 0.14285714 0.15714286 0.17142857 0.18571429 0.2 0.21428571 0.22857143 0.24285714 0.25714286 0.27142857 0.28571429 0.3 0.31428571 0.32857143 0.34285714 0.35714286 0.37142857 0.38571429 0.4 0.41428571 0.42857143 0.44285714 0.45714286 0.47142857 0.48571429 0.5 0.51428571 0.52857143 0.54285714 0.55714286 0.57142857 0.58571429 0.6 0.61428571 0.62857143 0.64285714 0.65714286 0.67142857 0.68571429 0.7 0.71428571 0.72857143 0.74285714 0.75714286 0.77142857 0.78571429 0.8 0.81428571 0.82857143 0.84285714 0.85714286 0.87142857 0.88571429 0.9 0.91428571 0.92857143 0.94285714 0.95714286 0.97142857 0.98571429 1 1 1 1 1 1
  arc A14 (-3.1035, -69.9312) -> (3.1035, -69.9312) centre (0, 0) ccw
  spline S7 degree 5 poles (3.1035, -69.9312) (3.1292, -69.8928) (3.1804, -69.816) (3.2569, -69.7008) (3.3581, -69.5468) (3.4834, -69.354) (3.6073, -69.1607) (3.73, -68.967) (3.8514, -68.7729) (3.9715, -68.5784) (4.0902, -68.3835) (4.2077, -68.1883) (4.3238, -67.9926) (4.4385, -67.7965) (4.552, -67.6001) (4.664, -67.4033) (4.7747, -67.2061) (4.884, -67.0085) (4.9919, -66.8106) (5.0984, -66.6124) (5.2035, -66.4138) (5.3071, -66.2148) (5.4094, -66.0155) (5.5101, -65.8159) (5.6095, -65.616) (5.7073, -65.4157) (5.8037, -65.2151) (5.8985, -65.0142) (5.9919, -64.813) (6.0837, -64.6115) (6.174, -64.4097) (6.2628, -64.2077) (6.3499, -64.0053) (6.4355, -63.8027) (6.5195, -63.5998) (6.6018, -63.3967) (6.6825, -63.1933) (6.7616, -62.9896) (6.839, -62.7857) (6.9148, -62.5816) (6.9888, -62.3773) (7.061, -62.1727) (7.1315, -61.9679) (7.2001, -61.7629) (7.267, -61.5578) (7.332, -61.3524) (7.3952, -61.1469) (7.4565, -60.9412) (7.516, -60.7353) (7.5736, -60.5293) (7.6291, -60.3231) (7.6825, -60.1168) (7.7337, -59.9104) (7.7827, -59.7039) (7.8293, -59.4973) (7.8739, -59.2907) (7.9164, -59.0839) (7.957, -58.877) (7.9955, -58.6701) (8.0317, -58.4632) (8.0651, -58.2562) (8.0952, -58.0493) (8.1217, -57.8425) (8.1445, -57.6357) (8.1642, -57.429) (8.1814, -57.2224) (8.1967, -57.0158) (8.2105, -56.8094) (8.2218, -56.6031) (8.2288, -56.3971) (8.2285, -56.1916) (8.2201, -56.0278) (8.2082, -55.9054) (8.1975, -55.824) (8.1916, -55.7833) knots -1 -1 -1 -1 -1 -1 -0.98571429 -0.97142857 -0.95714286 -0.94285714 -0.92857143 -0.91428571 -0.9 -0.88571429 -0.87142857 -0.85714286 -0.84285714 -0.82857143 -0.81428571 -0.8 -0.78571429 -0.77142857 -0.75714286 -0.74285714 -0.72857143 -0.71428571 -0.7 -0.68571429 -0.67142857 -0.65714286 -0.64285714 -0.62857143 -0.61428571 -0.6 -0.58571429 -0.57142857 -0.55714286 -0.54285714 -0.52857143 -0.51428571 -0.5 -0.48571429 -0.47142857 -0.45714286 -0.44285714 -0.42857143 -0.41428571 -0.4 -0.38571429 -0.37142857 -0.35714286 -0.34285714 -0.32857143 -0.31428571 -0.3 -0.28571429 -0.27142857 -0.25714286 -0.24285714 -0.22857143 -0.21428571 -0.2 -0.18571429 -0.17142857 -0.15714286 -0.14285714 -0.12857143 -0.11428571 -0.1 -0.08571429 -0.07142857 -0.05714286 -0.04285714 -0.02857143 -0.01428571 0 0 0 0 0 0
  line L7 (8.1916, -55.7833) -> (7.3211, -49.8557)
  arc A15 (8.9311, -47.5994) -> (7.3211, -49.8557) centre (9.2999, -49.5651) ccw
  arc A16 (8.9311, -47.5994) -> (16.0652, -45.6878) centre (0, 0) ccw
  arc A17 (18.5876, -46.8368) -> (16.0652, -45.6878) centre (16.7286, -47.5746) ccw
  line L8 (18.5876, -46.8368) -> (20.7976, -52.4056)
  spline S8 degree 5 poles (20.7976, -52.4056) (20.8127, -52.4438) (20.8442, -52.5196) (20.8951, -52.6316) (20.9697, -52.7776) (21.0722, -52.9557) (21.1812, -53.1306) (21.2942, -53.3036) (21.4093, -53.4755) (21.5259, -53.6467) (21.6441, -53.8171) (21.7645, -53.9863) (21.8876, -54.1539) (22.014, -54.3198) (22.1436, -54.4839) (22.276, -54.6464) (22.4108, -54.8076) (22.5476, -54.9675) (22.6861, -55.1264) (22.8264, -55.2842) (22.9683, -55.4409) (23.112, -55.5965) (23.2576, -55.7508) (23.4052, -55.904) (23.5546, -56.0559) (23.7057, -56.2067) (23.8586, -56.3563) (24.0131, -56.5049) (24.1691, -56.6523) (24.3265, -56.7987) (24.4855, -56.9441) (24.646, -57.0884) (24.8079, -57.2315) (24.9713, -57.3736) (25.1362, -57.5147) (25.3024, -57.6546) (25.4701, -57.7936) (25.6391, -57.9314) (25.8094, -58.0682) (25.981, -58.204) (26.1539, -58.3388) (26.328, -58.4725) (26.5035, -58.6052) (26.6801, -58.7369) (26.858, -58.8675) (27.0371, -58.9971) (27.2174, -59.1257) (27.3988, -59.2532) (27.5814, -59.3798) (27.7652, -59.5053) (27.95, -59.6298) (28.136, -59.7533) (28.3231, -59.8758) (28.5113, -59.9973) (28.7005, -60.1177) (28.8909, -60.2372) (29.0822, -60.3556) (29.2746, -60.4731) (29.468, -60.5895) (29.6625, -60.7049) (29.8579, -60.8194) (30.0544, -60.9328) (30.2518, -61.0452) (30.4502, -61.1566) (30.6495, -61.267) (30.8498, -61.3764) (31.0511, -61.4848) (31.2532, -61.5922) (31.4563, -61.6986) (31.6603, -61.804) (31.8652, -61.9084) (32.0298, -61.9911) (32.1537, -62.0527) (32.2365, -62.0935) (32.2779, -62.1139) knots 0 0 0 0 0 0 0.01428571 0.02857143 0.04285714 0.05714286 0.07142857 0.08571429 0.1 0.11428571 0.12857143 0.14285714 0.15714286 0.17142857 0.18571429 0.2 0.21428571 0.22857143 0.24285714 0.25714286 0.27142857 0.28571429 0.3 0.31428571 0.32857143 0.34285714 0.35714286 0.37142857 0.38571429 0.4 0.41428571 0.42857143 0.44285714 0.45714286 0.47142857 0.48571429 0.5 0.51428571 0.52857143 0.54285714 0.55714286 0.57142857 0.58571429 0.6 0.61428571 0.62857143 0.64285714 0.65714286 0.67142857 0.68571429 0.7 0.71428571 0.72857143 0.74285714 0.75714286 0.77142857 0.78571429 0.8 0.81428571 0.82857143 0.84285714 0.85714286 0.87142857 0.88571429 0.9 0.91428571 0.92857143 0.94285714 0.95714286 0.97142857 0.98571429 1 1 1 1 1 1
  arc A18 (32.2779, -62.1139) -> (37.6533, -59.0104) centre (0, 0) ccw
  spline S9 degree 5 poles (37.6533, -59.0104) (37.6563, -58.9644) (37.6623, -58.8723) (37.6709, -58.7342) (37.6816, -58.5502) (37.6937, -58.3206) (37.7044, -58.0913) (37.7138, -57.8622) (37.7219, -57.6334) (37.7286, -57.4049) (37.734, -57.1768) (37.7381, -56.9489) (37.7408, -56.7214) (37.7421, -56.4942) (37.7421, -56.2674) (37.7408, -56.0409) (37.738, -55.8148) (37.7339, -55.5891) (37.7284, -55.3638) (37.7215, -55.1388) (37.7132, -54.9143) (37.7035, -54.6901) (37.6924, -54.4664) (37.6799, -54.2432) (37.6659, -54.0204) (37.6505, -53.798) (37.6337, -53.5761) (37.6154, -53.3547) (37.5957, -53.1338) (37.5744, -52.9134) (37.5517, -52.6935) (37.5276, -52.4741) (37.5019, -52.2553) (37.4747, -52.037) (37.4459, -51.8193) (37.4157, -51.6022) (37.3839, -51.3857) (37.3505, -51.1698) (37.3156, -50.9545) (37.2792, -50.7399) (37.2411, -50.5259) (37.2014, -50.3126) (37.16, -50.1) (37.117, -49.8882) (37.0723, -49.6771) (37.0259, -49.4668) (36.9778, -49.2572) (36.9281, -49.0484) (36.8767, -48.8403) (36.8235, -48.6331) (36.7686, -48.4268) (36.7117, -48.2214) (36.6528, -48.0171) (36.5919, -47.8138) (36.5291, -47.6115) (36.4643, -47.4103) (36.3978, -47.2099) (36.3295, -47.0105) (36.2594, -46.8121) (36.1872, -46.6148) (36.1127, -46.4188) (36.0353, -46.2246) (35.9548, -46.0322) (35.8712, -45.8417) (35.7849, -45.6529) (35.6965, -45.4654) (35.6065, -45.2788) (35.5151, -45.0931) (35.4218, -44.9088) (35.3249, -44.7269) (35.2219, -44.5491) (35.1327, -44.4115) (35.0612, -44.3114) (35.0113, -44.2462) (34.9858, -44.214) knots -1 -1 -1 -1 -1 -1 -0.98571429 -0.97142857 -0.95714286 -0.94285714 -0.92857143 -0.91428571 -0.9 -0.88571429 -0.87142857 -0.85714286 -0.84285714 -0.82857143 -0.81428571 -0.8 -0.78571429 -0.77142857 -0.75714286 -0.74285714 -0.72857143 -0.71428571 -0.7 -0.68571429 -0.67142857 -0.65714286 -0.64285714 -0.62857143 -0.61428571 -0.6 -0.58571429 -0.57142857 -0.55714286 -0.54285714 -0.52857143 -0.51428571 -0.5 -0.48571429 -0.47142857 -0.45714286 -0.44285714 -0.42857143 -0.41428571 -0.4 -0.38571429 -0.37142857 -0.35714286 -0.34285714 -0.32857143 -0.31428571 -0.3 -0.28571429 -0.27142857 -0.25714286 -0.24285714 -0.22857143 -0.21428571 -0.2 -0.18571429 -0.17142857 -0.15714286 -0.14285714 -0.12857143 -0.11428571 -0.1 -0.08571429 -0.07142857 -0.05714286 -0.04285714 -0.02857143 -0.01428571 0 0 0 0 0 0
  line L9 (34.9858, -44.214) -> (31.2681, -39.5157)
  arc A19 (31.5342, -36.7567) -> (31.2681, -39.5157) centre (32.8365, -38.2747) ccw
  arc A20 (31.5342, -36.7567) -> (36.7567, -31.5342) centre (0, 0) ccw
  arc A21 (39.5157, -31.2681) -> (36.7567, -31.5342) centre (38.2747, -32.8365) ccw
  line L10 (39.5157, -31.2681) -> (44.214, -34.9858)
  spline S10 degree 5 poles (44.214, -34.9858) (44.2462, -35.0113) (44.3114, -35.0612) (44.4115, -35.1327) (44.5491, -35.2219) (44.7269, -35.3249) (44.9088, -35.4218) (45.0931, -35.5151) (45.2788, -35.6065) (45.4654, -35.6965) (45.6529, -35.7849) (45.8417, -35.8712) (46.0322, -35.9548) (46.2246, -36.0353) (46.4188, -36.1127) (46.6148, -36.1872) (46.8121, -36.2594) (47.0105, -36.3295) (47.2099, -36.3978) (47.4103, -36.4643) (47.6115, -36.5291) (47.8138, -36.5919) (48.0171, -36.6528) (48.2214, -36.7117) (48.4268, -36.7686) (48.6331, -36.8235) (48.8403, -36.8767) (49.0484, -36.9281) (49.2572, -36.9778) (49.4668, -37.0259) (49.6771, -37.0723) (49.8882, -37.117) (50.1, -37.16) (50.3126, -37.2014) (50.5259, -37.2411) (50.7399, -37.2792) (50.9545, -37.3156) (51.1698, -37.3505) (51.3857, -37.3839) (51.6022, -37.4157) (51.8193, -37.4459) (52.037, -37.4747) (52.2553, -37.5019) (52.4741, -37.5276) (52.6935, -37.5517) (52.9134, -37.5744) (53.1338, -37.5957) (53.3547, -37.6154) (53.5761, -37.6337) (53.798, -37.6505) (54.0204, -37.6659) (54.2432, -37.6799) (54.4664, -37.6924) (54.6901, -37.7035) (54.9143, -37.7132) (55.1388, -37.7215) (55.3638, -37.7284) (55.5891, -37.7339) (55.8148, -37.738) (56.0409, -37.7408) (56.2674, -37.7421) (56.4942, -37.7421) (56.7214, -37.7408) (56.9489, -37.7381) (57.1768, -37.734) (57.4049, -37.7286) (57.6334, -37.7219) (57.8622, -37.7138) (58.0913, -37.7044) (58.3206, -37.6937) (58.5502, -37.6816) (58.7342, -37.6709) (58.8723, -37.6623) (58.9644, -37.6563) (59.0104, -37.6533) knots 0 0 0 0 0 0 0.01428571 0.02857143 0.04285714 0.05714286 0.07142857 0.08571429 0.1 0.11428571 0.12857143 0.14285714 0.15714286 0.17142857 0.18571429 0.2 0.21428571 0.22857143 0.24285714 0.25714286 0.27142857 0.28571429 0.3 0.31428571 0.32857143 0.34285714 0.35714286 0.37142857 0.38571429 0.4 0.41428571 0.42857143 0.44285714 0.45714286 0.47142857 0.48571429 0.5 0.51428571 0.52857143 0.54285714 0.55714286 0.57142857 0.58571429 0.6 0.61428571 0.62857143 0.64285714 0.65714286 0.67142857 0.68571429 0.7 0.71428571 0.72857143 0.74285714 0.75714286 0.77142857 0.78571429 0.8 0.81428571 0.82857143 0.84285714 0.85714286 0.87142857 0.88571429 0.9 0.91428571 0.92857143 0.94285714 0.95714286 0.97142857 0.98571429 1 1 1 1 1 1
  arc A22 (59.0104, -37.6533) -> (62.1139, -32.2779) centre (0, 0) ccw
  spline S11 degree 5 poles (62.1139, -32.2779) (62.0935, -32.2365) (62.0527, -32.1537) (61.9911, -32.0298) (61.9084, -31.8652) (61.804, -31.6603) (61.6986, -31.4563) (61.5922, -31.2532) (61.4848, -31.0511) (61.3764, -30.8498) (61.267, -30.6495) (61.1566, -30.4502) (61.0452, -30.2518) (60.9328, -30.0544) (60.8194, -29.8579) (60.7049, -29.6625) (60.5895, -29.468) (60.4731, -29.2746) (60.3556, -29.0822) (60.2372, -28.8909) (60.1177, -28.7005) (59.9973, -28.5113) (59.8758, -28.3231) (59.7533, -28.136) (59.6298, -27.95) (59.5053, -27.7652) (59.3798, -27.5814) (59.2532, -27.3988) (59.1257, -27.2174) (58.9971, -27.0371) (58.8675, -26.858) (58.7369, -26.6801) (58.6052, -26.5035) (58.4725, -26.328) (58.3388, -26.1539) (58.204, -25.981) (58.0682, -25.8094) (57.9314, -25.6391) (57.7936, -25.4701) (57.6546, -25.3024) (57.5147, -25.1362) (57.3736, -24.9713) (57.2315, -24.8079) (57.0884, -24.646) (56.9441, -24.4855) (56.7987, -24.3265) (56.6523, -24.1691) (56.5049, -24.0131) (56.3563, -23.8586) (56.2067, -23.7057) (56.0559, -23.5546) (55.904, -23.4052) (55.7508, -23.2576) (55.5965, -23.112) (55.4409, -22.9683) (55.2842, -22.8264) (55.1264, -22.6861) (54.9675, -22.5476) (54.8076, -22.4108) (54.6464, -22.276) (54.4839, -22.1436) (54.3198, -22.014) (54.1539, -21.8876) (53.9863, -21.7645) (53.8171, -21.6441) (53.6467, -21.5259) (53.4755, -21.4093) (53.3036, -21.2942) (53.1306, -21.1812) (52.9557, -21.0722) (52.7776, -20.9697) (52.6316, -20.8951) (52.5196, -20.8442) (52.4438, -20.8127) (52.4056, -20.7976) knots -1 -1 -1 -1 -1 -1 -0.98571429 -0.97142857 -0.95714286 -0.94285714 -0.92857143 -0.91428571 -0.9 -0.88571429 -0.87142857 -0.85714286 -0.84285714 -0.82857143 -0.81428571 -0.8 -0.78571429 -0.77142857 -0.75714286 -0.74285714 -0.72857143 -0.71428571 -0.7 -0.68571429 -0.67142857 -0.65714286 -0.64285714 -0.62857143 -0.61428571 -0.6 -0.58571429 -0.57142857 -0.55714286 -0.54285714 -0.52857143 -0.51428571 -0.5 -0.48571429 -0.47142857 -0.45714286 -0.44285714 -0.42857143 -0.41428571 -0.4 -0.38571429 -0.37142857 -0.35714286 -0.34285714 -0.32857143 -0.31428571 -0.3 -0.28571429 -0.27142857 -0.25714286 -0.24285714 -0.22857143 -0.21428571 -0.2 -0.18571429 -0.17142857 -0.15714286 -0.14285714 -0.12857143 -0.11428571 -0.1 -0.08571429 -0.07142857 -0.05714286 -0.04285714 -0.02857143 -0.01428571 0 0 0 0 0 0
  line L11 (52.4056, -20.7976) -> (46.8368, -18.5876)
  arc A23 (45.6878, -16.0652) -> (46.8368, -18.5876) centre (47.5746, -16.7286) ccw
  arc A24 (45.6878, -16.0652) -> (47.5994, -8.9311) centre (0, 0) ccw
  arc A25 (49.8557, -7.3211) -> (47.5994, -8.9311) centre (49.5651, -9.2999) ccw
  line L12 (49.8557, -7.3211) -> (55.7833, -8.1916)
  spline S12 degree 5 poles (55.7833, -8.1916) (55.824, -8.1975) (55.9054, -8.2082) (56.0278, -8.2201) (56.1916, -8.2285) (56.3971, -8.2288) (56.6031, -8.2218) (56.8094, -8.2105) (57.0158, -8.1967) (57.2224, -8.1814) (57.429, -8.1642) (57.6357, -8.1445) (57.8425, -8.1217) (58.0493, -8.0952) (58.2562, -8.0651) (58.4632, -8.0317) (58.6701, -7.9955) (58.877, -7.957) (59.0839, -7.9164) (59.2907, -7.8739) (59.4973, -7.8293) (59.7039, -7.7827) (59.9104, -7.7337) (60.1168, -7.6825) (60.3231, -7.6291) (60.5293, -7.5736) (60.7353, -7.516) (60.9412, -7.4565) (61.1469, -7.3952) (61.3524, -7.332) (61.5578, -7.267) (61.7629, -7.2001) (61.9679, -7.1315) (62.1727, -7.061) (62.3773, -6.9888) (62.5816, -6.9148) (62.7857, -6.839) (62.9896, -6.7616) (63.1933, -6.6825) (63.3967, -6.6018) (63.5998, -6.5195) (63.8027, -6.4355) (64.0053, -6.3499) (64.2077, -6.2628) (64.4097, -6.174) (64.6115, -6.0837) (64.813, -5.9919) (65.0142, -5.8985) (65.2151, -5.8037) (65.4157, -5.7073) (65.616, -5.6095) (65.8159, -5.5101) (66.0155, -5.4094) (66.2148, -5.3071) (66.4138, -5.2035) (66.6124, -5.0984) (66.8106, -4.9919) (67.0085, -4.884) (67.2061, -4.7747) (67.4033, -4.664) (67.6001, -4.552) (67.7965, -4.4385) (67.9926, -4.3238) (68.1883, -4.2077) (68.3835, -4.0902) (68.5784, -3.9715) (68.7729, -3.8514) (68.967, -3.73) (69.1607, -3.6073) (69.354, -3.4834) (69.5468, -3.3581) (69.7008, -3.2569) (69.816, -3.1804) (69.8928, -3.1292) (69.9312, -3.1035) knots 0 0 0 0 0 0 0.01428571 0.02857143 0.04285714 0.05714286 0.07142857 0.08571429 0.1 0.11428571 0.12857143 0.14285714 0.15714286 0.17142857 0.18571429 0.2 0.21428571 0.22857143 0.24285714 0.25714286 0.27142857 0.28571429 0.3 0.31428571 0.32857143 0.34285714 0.35714286 0.37142857 0.38571429 0.4 0.41428571 0.42857143 0.44285714 0.45714286 0.47142857 0.48571429 0.5 0.51428571 0.52857143 0.54285714 0.55714286 0.57142857 0.58571429 0.6 0.61428571 0.62857143 0.64285714 0.65714286 0.67142857 0.68571429 0.7 0.71428571 0.72857143 0.74285714 0.75714286 0.77142857 0.78571429 0.8 0.81428571 0.82857143 0.84285714 0.85714286 0.87142857 0.88571429 0.9 0.91428571 0.92857143 0.94285714 0.95714286 0.97142857 0.98571429 1 1 1 1 1 1
  arc A26 (69.9312, -3.1035) -> (69.9312, 3.1035) centre (0, 0) ccw
  spline S13 degree 5 poles (69.9312, 3.1035) (69.8928, 3.1292) (69.816, 3.1804) (69.7008, 3.2569) (69.5468, 3.3581) (69.354, 3.4834) (69.1607, 3.6073) (68.967, 3.73) (68.7729, 3.8514) (68.5784, 3.9715) (68.3835, 4.0902) (68.1883, 4.2077) (67.9926, 4.3238) (67.7965, 4.4385) (67.6001, 4.552) (67.4033, 4.664) (67.2061, 4.7747) (67.0085, 4.884) (66.8106, 4.9919) (66.6124, 5.0984) (66.4138, 5.2035) (66.2148, 5.3071) (66.0155, 5.4094) (65.8159, 5.5101) (65.616, 5.6095) (65.4157, 5.7073) (65.2151, 5.8037) (65.0142, 5.8985) (64.813, 5.9919) (64.6115, 6.0837) (64.4097, 6.174) (64.2077, 6.2628) (64.0053, 6.3499) (63.8027, 6.4355) (63.5998, 6.5195) (63.3967, 6.6018) (63.1933, 6.6825) (62.9896, 6.7616) (62.7857, 6.839) (62.5816, 6.9148) (62.3773, 6.9888) (62.1727, 7.061) (61.9679, 7.1315) (61.7629, 7.2001) (61.5578, 7.267) (61.3524, 7.332) (61.1469, 7.3952) (60.9412, 7.4565) (60.7353, 7.516) (60.5293, 7.5736) (60.3231, 7.6291) (60.1168, 7.6825) (59.9104, 7.7337) (59.7039, 7.7827) (59.4973, 7.8293) (59.2907, 7.8739) (59.0839, 7.9164) (58.877, 7.957) (58.6701, 7.9955) (58.4632, 8.0317) (58.2562, 8.0651) (58.0493, 8.0952) (57.8425, 8.1217) (57.6357, 8.1445) (57.429, 8.1642) (57.2224, 8.1814) (57.0158, 8.1967) (56.8094, 8.2105) (56.6031, 8.2218) (56.3971, 8.2288) (56.1916, 8.2285) (56.0278, 8.2201) (55.9054, 8.2082) (55.824, 8.1975) (55.7833, 8.1916) knots -1 -1 -1 -1 -1 -1 -0.98571429 -0.97142857 -0.95714286 -0.94285714 -0.92857143 -0.91428571 -0.9 -0.88571429 -0.87142857 -0.85714286 -0.84285714 -0.82857143 -0.81428571 -0.8 -0.78571429 -0.77142857 -0.75714286 -0.74285714 -0.72857143 -0.71428571 -0.7 -0.68571429 -0.67142857 -0.65714286 -0.64285714 -0.62857143 -0.61428571 -0.6 -0.58571429 -0.57142857 -0.55714286 -0.54285714 -0.52857143 -0.51428571 -0.5 -0.48571429 -0.47142857 -0.45714286 -0.44285714 -0.42857143 -0.41428571 -0.4 -0.38571429 -0.37142857 -0.35714286 -0.34285714 -0.32857143 -0.31428571 -0.3 -0.28571429 -0.27142857 -0.25714286 -0.24285714 -0.22857143 -0.21428571 -0.2 -0.18571429 -0.17142857 -0.15714286 -0.14285714 -0.12857143 -0.11428571 -0.1 -0.08571429 -0.07142857 -0.05714286 -0.04285714 -0.02857143 -0.01428571 0 0 0 0 0 0
  line L13 (55.7833, 8.1916) -> (49.8557, 7.3211)
  arc A27 (47.5994, 8.9311) -> (49.8557, 7.3211) centre (49.5651, 9.2999) ccw
  arc A28 (47.5994, 8.9311) -> (45.6878, 16.0652) centre (0, 0) ccw
  arc A29 (46.8368, 18.5876) -> (45.6878, 16.0652) centre (47.5746, 16.7286) ccw
  line L14 (46.8368, 18.5876) -> (52.4056, 20.7976)
  spline S14 degree 5 poles (52.4056, 20.7976) (52.4438, 20.8127) (52.5196, 20.8442) (52.6316, 20.8951) (52.7776, 20.9697) (52.9557, 21.0722) (53.1306, 21.1812) (53.3036, 21.2942) (53.4755, 21.4093) (53.6467, 21.5259) (53.8171, 21.6441) (53.9863, 21.7645) (54.1539, 21.8876) (54.3198, 22.014) (54.4839, 22.1436) (54.6464, 22.276) (54.8076, 22.4108) (54.9675, 22.5476) (55.1264, 22.6861) (55.2842, 22.8264) (55.4409, 22.9683) (55.5965, 23.112) (55.7508, 23.2576) (55.904, 23.4052) (56.0559, 23.5546) (56.2067, 23.7057) (56.3563, 23.8586) (56.5049, 24.0131) (56.6523, 24.1691) (56.7987, 24.3265) (56.9441, 24.4855) (57.0884, 24.646) (57.2315, 24.8079) (57.3736, 24.9713) (57.5147, 25.1362) (57.6546, 25.3024) (57.7936, 25.4701) (57.9314, 25.6391) (58.0682, 25.8094) (58.204, 25.981) (58.3388, 26.1539) (58.4725, 26.328) (58.6052, 26.5035) (58.7369, 26.6801) (58.8675, 26.858) (58.9971, 27.0371) (59.1257, 27.2174) (59.2532, 27.3988) (59.3798, 27.5814) (59.5053, 27.7652) (59.6298, 27.95) (59.7533, 28.136) (59.8758, 28.3231) (59.9973, 28.5113) (60.1177, 28.7005) (60.2372, 28.8909) (60.3556, 29.0822) (60.4731, 29.2746) (60.5895, 29.468) (60.7049, 29.6625) (60.8194, 29.8579) (60.9328, 30.0544) (61.0452, 30.2518) (61.1566, 30.4502) (61.267, 30.6495) (61.3764, 30.8498) (61.4848, 31.0511) (61.5922, 31.2532) (61.6986, 31.4563) (61.804, 31.6603) (61.9084, 31.8652) (61.9911, 32.0298) (62.0527, 32.1537) (62.0935, 32.2365) (62.1139, 32.2779) knots 0 0 0 0 0 0 0.01428571 0.02857143 0.04285714 0.05714286 0.07142857 0.08571429 0.1 0.11428571 0.12857143 0.14285714 0.15714286 0.17142857 0.18571429 0.2 0.21428571 0.22857143 0.24285714 0.25714286 0.27142857 0.28571429 0.3 0.31428571 0.32857143 0.34285714 0.35714286 0.37142857 0.38571429 0.4 0.41428571 0.42857143 0.44285714 0.45714286 0.47142857 0.48571429 0.5 0.51428571 0.52857143 0.54285714 0.55714286 0.57142857 0.58571429 0.6 0.61428571 0.62857143 0.64285714 0.65714286 0.67142857 0.68571429 0.7 0.71428571 0.72857143 0.74285714 0.75714286 0.77142857 0.78571429 0.8 0.81428571 0.82857143 0.84285714 0.85714286 0.87142857 0.88571429 0.9 0.91428571 0.92857143 0.94285714 0.95714286 0.97142857 0.98571429 1 1 1 1 1 1
  arc A30 (62.1139, 32.2779) -> (59.0104, 37.6533) centre (0, 0) ccw